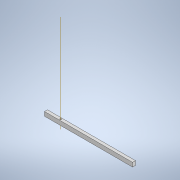
# Autodesk Inventor part: Grua Maya
Saved by Autodesk Inventor 2020 (Build 240168000, 168)
## iProperties
Created: 2019-10-05
Part Number: Grua Maya
Material: Genérico
Document SubType Name: Modeling
Designer: dasa1
Density: 1 g/cm^3
Appearance: Valor por defecto
Author: dasa1
Autodesk Inventor part; units mm, degrees
ref_plane "YZ Plane" through (0, 0, 0) normal (1, 0, 0) x (0, 1, 0)
ref_plane "XZ Plane" through (0, 0, 0) normal (0, 1, 0) x (-1, 0, 0)
ref_plane "XY Plane" through (0, 0, 0) normal (0, 0, 1) x (1, 0, 0)
sketch "Boceto1" plane through (0, 0, 0) normal (0, 1, 0) x (-1, 0, 0)
  line L0 (0, 0) -> (500, 0) construction
  line L1 (500, 0) -> (500, -50) construction
  line L2 (500, -50) -> (0, -50) construction
  line L3 (0, -50) -> (0, 0) construction
  line L4 (500, -50) -> (-2500, -50)
  line L5 (-2500, -50) -> (-2500, 50)
  line L6 (-2500, 50) -> (500, 50)
  line L7 (500, 50) -> (500, -50)
  circle A0 centre (0, 0) radius 25
  dimension "d0" = 500
  dimension "d1" = 50
  dimension "d2" = 3000
  dimension "d3" = 100
  dimension "d16" = 50
  constraints: 16 end point, 4 parallel, 2 horizontal, 2 perpendicular, 1 centre point, 1 coincident
  measures "d0" distance of L1.end L2.end
  measures "d1" distance of L0.end L1.end
  measures "d2" distance of L5.end L6.end
  measures "d3" distance of L4.end L5.end
  measures "d16" diameter of A0
extrude "Extrusión1" add sketch "Boceto1" along normal blind 140 contours L4 L5 L6 L7 | A0
chamfer "Chaflán1" [suppressed]
sketch "Boceto2" plane through (0, 0, 0) normal (0, -1, 0) x (1, 0, 0)
  line L0 (-500, -50) -> (-500, 50) construction
  line L1 (-500, 50) -> (0, 50) construction
  line L2 (0, 50) -> (0, 0) construction
  line L3 (0, 0) -> (-500, 0) construction
  line L4 (-500, 0) -> (-500, 50) construction
  circle A0 centre (0, 0) radius 25
  point P0 (0, 0)
  dimension "d17" = 50
  dimension "d18" = 500
  dimension "d19" = 50
  constraints: 8 end point, 2 parallel, 1 centre point, 1 coincident, 1 horizontal, 1 perpendicular
  measures "d17" diameter of A0
  measures "d18" distance between parallel lines of L2 L0
  measures "d19" distance between parallel lines of L1 L3
hole "Agujero1" at (0, 0, 0) direction (0, 1, 0) diameter 50 end through all
ref_plane "Plano de trabajo1" through (0, 3004.9293, 0) normal (0, 0, 1) x (0, -1, 0)
sketch "Boceto3" plane through (0, 3004.9293, 0) normal (0, 0, 1) x (0, -1, 0)
  line L0 (3004.9293, 0) -> (2145.9293, 0) construction
  ellipse E0 centre (2864.9293, 0) end of major axis (2933.6162, 0) minor radius 25 (2864.9293, -25) -> (2864.9293, 25) ccw construction
  line L1 (2864.9293, 2450) -> (3002.3032, 2500) construction
  line L2 (2864.9293, 2450) -> (2864.9293, 1950) construction
  line L3 (2864.9293, 25) -> (2864.9293, 2450) construction
  line L4 (2145.9293, 0) -> (2153.9293, 0)
  line L5 (2153.9293, -9) -> (2153.9293, -15)
  line L6 (2149.9293, -15) -> (2149.9293, -15)
  line L7 (2145.9293, -11) -> (2145.9293, -9)
  line L8 (2145.9293, -15) -> (2153.9293, -15)
  line L9 (2153.9293, -11) -> (2153.9293, -5)
  line L10 (2149.9293, -5) -> (2149.9293, -5)
  line L11 (2145.9293, -5) -> (2145.9293, -15)
  arc A0 (2145.9293, -11) -> (2149.9293, -15) centre (2149.9293, -11) ccw
  arc A1 (2149.9293, -15) -> (2153.9293, -11) centre (2149.9293, -11) ccw
  arc A2 (2153.9293, -9) -> (2149.9293, -5) centre (2149.9293, -9) ccw
  arc A3 (2149.9293, -5) -> (2145.9293, -9) centre (2149.9293, -9) ccw
  circle A4 centre (2149.9293, -9) radius 4
  point P0 (2149.9293, -5)
  dimension "d20" = 859
  dimension "d21" = 500
  dimension "d22" = 8
  dimension "d23" = 15
  dimension "d24" = 10
  dimension "d25" = 4
  constraints: 20 end point, 10 point on line, 8 point on circle, 8 tangent, 4 centre point, 4 parallel, 3 equal radius, 3 horizontal, 2 perpendicular, 1 coincident, 4 other
  measures "d20" distance of L0.start L0.end
  measures "d21" distance of L1.start L2.end
  measures "d22" distance of L5.end L8.start
  measures "d23" distance of L4.end L5.end
  measures "d24" distance of L9.end L8.end
  measures "d25" radius of A0
revolve "Revolución1" [suppressed]
sketch "Boceto4" plane through (0, 3004.9293, 0) normal (0, 0, 1) x (0, -1, 0)
  line L0 (3004.9293, -500) -> (3004.9293, 2500) construction
  line L1 (3004.9293, 2500) -> (3004.9293, 2000) construction
  line L2 (3004.9293, 2000) -> (2864.9293, 2000) construction
  line L3 (2864.9293, 25) -> (2864.9293, 2450) construction
  line L4 (2864.9293, 2000) -> (2145.9293, 9)
  arc A0 (2153.9293, 9) -> (2145.9293, 9) centre (2149.9293, 9) ccw projected
  line L5 (2153.9293, 9) -> (2864.9293, 1977.4084)
  line L6 (2153.9293, 9) -> (4246.8107, 9) construction
  line L7 (2864.9293, 1977.4084) -> (2864.9293, 2000)
  line L8 (2149.9293, 9) -> (2864.9293, 1988.4824)
  line L9 (2149.9293, 9) -> (4254.585, 9) construction
  point P0 (3004.9293, 0)
  point P1 (2146.8522, 11.5557)
  point P2 (2151.2882, 12.7621)
  dimension "d27" = 500
  dimension "d28" = 70.14
  dimension "d31" = 70.14
  constraints: 16 end point, 3 point on line, 2 equal length, 2 horizontal, 2 point on circle, 1 collinear, 1 perpendicular
  measures "d27" distance of L0.end L1.end
  measures "d28" angle of L6 L5
  measures "d31" angle of L9 L8
revolve "Revolución2" [suppressed]
